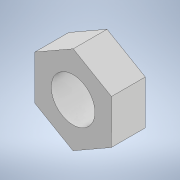
# Autodesk Inventor part: m4nut
Saved by Autodesk Inventor 2021 (Build 250183000, 183)
## iProperties
Created: 2024-04-26
Part Number: m4nut
Material: Generic
Document SubType Name: Modeling
Designer: Toby
Density: 1 g/cm^3
Appearance: Default
Author: Toby
Autodesk Inventor part; units mm, degrees
ref_plane "YZ Plane" through (0, 0, 0) normal (1, 0, 0) x (0, 1, 0)
ref_plane "XZ Plane" through (0, 0, 0) normal (0, 1, 0) x (-1, 0, 0)
ref_plane "XY Plane" through (0, 0, 0) normal (0, 0, 1) x (1, 0, 0)
sketch "Sketch1" plane through (0, 0, 0) normal (0, 0, 1) x (1, 0, 0)
  line L0 (3.5, -2.0347) -> (-0.0121, -4.0484)
  line L1 (-0.0121, -4.0484) -> (-3.5121, -2.0137)
  line L2 (-3.5121, -2.0137) -> (-3.5, 2.0347)
  line L3 (-3.5, 2.0347) -> (0.0121, 4.0484)
  line L4 (0.0121, 4.0484) -> (3.5121, 2.0137)
  line L5 (3.5121, 2.0137) -> (3.5, -2.0347)
  circle A0 centre (0, 0) radius 2
  point P0 (3.5, 0)
  dimension "d0" = 3.5
  dimension "d1" = 4
  constraints: 12 end point, 2 coincident, 1 centre point, 13 other
  measures "d0" distance of point (0, 0) point (3.5, 0)
  measures "d1" diameter of A0
extrude "Extrusion1" add sketch "Sketch1" along normal blind 3.1
body "Solid1"
